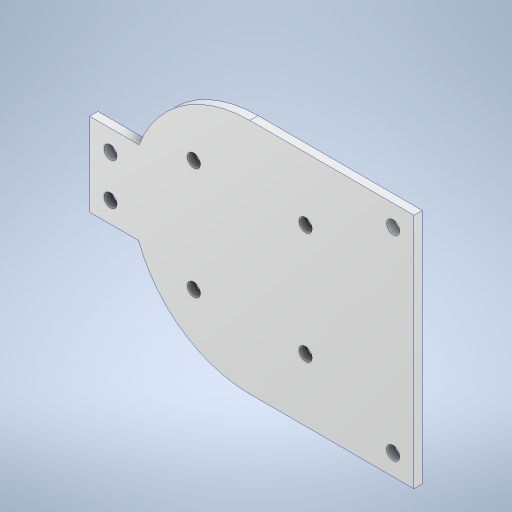
# Autodesk Inventor part: endeff_plate1
Saved by Autodesk Inventor 2024 (Build 280153000, 153)
## iProperties
Created: 2024-12-13
Part Number: endeff_plate1
Material: アルミニウム 6061
Document SubType Name: Modeling
Designer: hirek
Density: 2.7 g/cm^3
Appearance: アルミニウム - フラット
Mass: 15.4015 g
Surface Area: 62.3196 cm^2
Volume: 5.70425 cm^3
Author: hirek
Autodesk Inventor part; units mm, degrees
ref_plane "YZ Plane" through (0, 0, 0) normal (1, 0, 0) x (0, 1, 0)
ref_plane "XZ Plane" through (0, 0, 0) normal (0, 1, 0) x (-1, 0, 0)
ref_plane "XY Plane" through (0, 0, 0) normal (0, 0, 1) x (1, 0, 0)
sketch "スケッチ1" plane through (0, 0, 0) normal (0, 0, 1) x (1, 0, 0)
  circle A0 centre (0, 0) radius 28.5
  line L0 (0, 28.5) -> (39.5, 28.5)
  line L1 (39.5, 28.5) -> (39.5, -28.5)
  line L2 (39.5, -28.5) -> (0, -28.5)
  line L3 (0, -28.5) -> (0, 28.5)
  line L4 (0, 10.1136) -> (-38.5, 10.1136)
  line L5 (-38.5, 10.1136) -> (-38.5, -9.8864)
  line L6 (-38.5, -9.8864) -> (0, -9.8864)
  line L7 (0, -9.8864) -> (0, 10.1136)
  point P0 (28.5, 0)
  point P1 (-26.7303, -9.8864)
  point P2 (-26.6452, 10.1136)
  dimension "d0" = 57
  dimension "d19" = 39.5
  dimension "d38" = 38.5
  dimension "d39" = 20
  constraints: 16 end point, 4 parallel, 2 horizontal, 2 perpendicular, 1 coincident, 1 midpoint, 1 point on line, 3 other
  measures "d19" distance from line of L1 point (0, 0)
  measures "d38" distance of L6.end L5.end
  measures "d39" distance of L5.end L4.end
extrude "押し出し1" add sketch "スケッチ1" along normal blind 2
sketch "スケッチ3" plane through (0, 0, 2) normal (0, 0, 1) x (1, 0, 0)
  circle A0 centre (0, 0) radius 19
  line L0 (0, 0) -> (13.435, -13.435)
  line L1 (0, 0) -> (19, 0) construction
  line L2 (39.5, 28.5) -> (0, 28.5) projected
  line L3 (34.5, 28.5) -> (34.5, -28.5)
  line L4 (0, -28.5) -> (39.5, -28.5) projected
  line L5 (39.5, -28.5) -> (39.5, 28.5) projected
  line L6 (-26.6452, 10.1136) -> (-38.5, 10.1136) projected
  line L7 (-33.5, 10.1136) -> (-33.5, -9.8864)
  line L8 (-38.5, -9.8864) -> (-26.7303, -9.8864) projected
  line L9 (-38.5, 10.1136) -> (-38.5, -9.8864) projected
  point P0 (13.435, 13.435)
  point P1 (-13.435, 13.435)
  point P2 (-13.435, -13.435)
  point P3 (34.5, 23.5)
  point P4 (34.5, -23.5)
  point P5 (-33.5, 5.1136)
  point P6 (-33.5, -4.8864)
  point P7 (-32.6152, -9.8864)
  dimension "d22" = 38
  dimension "d23" = 45
  dimension "d26" = 360
  dimension "d28" = 5
  dimension "d29" = 5
  dimension "d37" = 5
  dimension "d40" = 5
  dimension "d41" = 5
  dimension "d42" = 5
  constraints: 8 end point, 8 point on line, 2 coincident, 2 vertical, 1 equal length, 1 horizontal, 1 midpoint, 8 other
  measures "d23" angle of L0 L1
  measures "d28" distance from line of point (34.5, 23.5) L2
  measures "d29" distance from line of L4 point (34.5, -23.5)
  measures "d37" distance between parallel lines of L5 L3
  measures "d40" distance from line of point (-33.5, 5.114) L6
  measures "d41" vertical distance of point (-32.615, -9.886) point (-33.5, -4.886)
  measures "d42" distance between parallel lines of L7 L9
hole "穴2" at (13.435, -13.435, 2) at (13.435, 13.435, 2) at (-13.435, 13.435, 2) at (-13.435, -13.435, 2) at (34.5, 23.5, 2) at (34.5, -23.5, 2) at (-33.5, 5.1136, 2) at (-33.5, -4.8864, 2) direction (0, 0, -1) diameter 3.2 end through all
